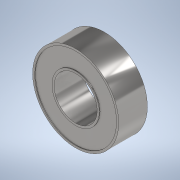
# Autodesk Inventor part: Rolamento 6x3x2mm
Saved by Autodesk Inventor 2021 (Build 250183000, 183)
## iProperties
Created: 2021-11-18
Part Number: Rolamento 6x3x2mm
Material: Generic
Document SubType Name: Modeling
Designer: Matheus
Density: 22.1049 g/cm^3
Appearance: Steel - Polished
Mass: 0.9 g
Surface Area: 1.01788 cm^2
Volume: 0.040715 cm^3
Author: Matheus
Autodesk Inventor part; units mm, degrees
ref_plane "YZ Plane" through (0, 0, 0) normal (1, 0, 0) x (0, 1, 0)
ref_plane "XZ Plane" through (0, 0, 0) normal (0, 1, 0) x (-1, 0, 0)
ref_plane "XY Plane" through (0, 0, 0) normal (0, 0, 1) x (1, 0, 0)
sketch "Sketch1" plane through (0, 0, 0) normal (1, 0, 0) x (0, 1, 0)
  line L0 (0, -1.4) -> (0, 1.4) construction
  line L1 (-0.6, 0) -> (3.6, 0) construction
  line L2 (1.65, 0.95) -> (2.85, 0.95)
  line L3 (2.85, 0.95) -> (2.85, 1)
  line L4 (2.85, 1) -> (3, 1)
  line L5 (3, 1) -> (3, -1)
  line L6 (3, -1) -> (2.85, -1)
  line L7 (2.85, -1) -> (2.85, -0.95)
  line L8 (2.85, -0.95) -> (1.65, -0.95)
  line L9 (1.5, 0.9) -> (1.5, -1)
  line L10 (1.5, 0.9) -> (1.5, 1)
  line L11 (1.5, 1) -> (1.65, 1)
  line L12 (1.65, 1) -> (1.65, 0.95)
  line L13 (1.5, -1) -> (1.65, -1)
  line L14 (1.65, -1) -> (1.65, -0.95)
  point P0 (0, 0)
  dimension "d0" = 3
  dimension "d1" = 6
  dimension "d2" = 0.15
  dimension "d3" = 0.05
  dimension "d4" = 2
  constraints: 26 end point, 7 perpendicular, 3 equal length, 3 symmetric about line, 2 point on line, 1 horizontal, 1 vertical, 1 other
  measures "d0" diameter of L9 L0
  measures "d1" diameter of L5 L0
  measures "d2" distance of L3.end L4.end
  measures "d3" distance of L2.end L3.end
  measures "d4" distance of L4.end L5.end
revolve "Revolution1" add sketch "Sketch1" angle 360 about axis through (0, 0, -10) along (0, 0, 1)
body "Solid1"
